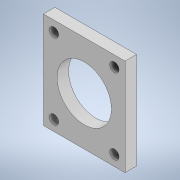
# Autodesk Inventor part: Placa cilindro hidraulico
Saved by Autodesk Inventor 2021 (Build 250183000, 183)
## iProperties
Created: 2021-07-12
Part Number: Placa cilindro hidraulico
Material: Generic
Document SubType Name: Modeling
Designer: Nelson
Density: 1 g/cm^3
Appearance: Default
Author: Nelson
Autodesk Inventor part; units mm, degrees
ref_plane "YZ Plane" through (0, 0, 0) normal (1, 0, 0) x (0, 1, 0)
ref_plane "XZ Plane" through (0, 0, 0) normal (0, 1, 0) x (-1, 0, 0)
ref_plane "XY Plane" through (0, 0, 0) normal (0, 0, 1) x (1, 0, 0)
sketch "Sketch1" plane through (0, 0, 0) normal (0, 0, 1) x (1, 0, 0)
  line L0 (0, 0) -> (270, 0)
  line L1 (0, 320) -> (0, 0)
  line L2 (270, 320) -> (0, 320)
  circle A0 centre (135, 160) radius 90
  circle A1 centre (35, 285) radius 15.25
  circle A2 centre (235, 285) radius 15.25
  circle A3 centre (235, 35) radius 15.25
  circle A4 centre (35, 35) radius 15.25
  line L3 (270, 0) -> (270, 320)
  point P0 (135, -160)
  dimension "d0" = 30.5
  dimension "d1" = 180
  dimension "d2" = 100
  dimension "d5" = 125
  dimension "d6" = 100
  dimension "d7" = 125
  dimension "d8" = 100
  dimension "d9" = 100
  dimension "d10" = 125
  dimension "d11" = 125
  dimension "d12" = 320
  dimension "d13" = 270
  dimension "d14" = 135
  dimension "d15" = 160
  constraints: 8 end point, 5 centre point, 2 equal radius, 1 coincident
  measures "d0" diameter of A1
  measures "d1" diameter of A0
  measures "d2" horizontal distance of A1.centre A0.centre
  measures "d5" vertical distance of A0.centre A1.centre
  measures "d6" horizontal distance of A0.centre A2.centre
  measures "d7" vertical distance of A0.centre A2.centre
  measures "d8" horizontal distance of A4.centre A0.centre
  measures "d9" horizontal distance of A3.centre A0.centre
  measures "d10" vertical distance of A0.centre A4.centre
  measures "d11" vertical distance of A3.centre A0.centre
  measures "d12" distance of L0.end L2.start
  measures "d13" distance of L0.start L0.end
  measures "d14" distance from line of L1 A0.centre
  measures "d15" distance from line of L2 A0.centre
extrude "Extrusion1" add sketch "Sketch1" against normal blind 38
equation "\"d6\" = d2"
equation "\"d7\" = d5"
equation "\"d8\" = d2"
equation "\"d9\" = d2"
equation "\"d10\" = d5"
equation "\"d11\" = d5"
body "Solid1"
